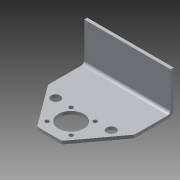
# Autodesk Inventor part: bracket for PG-71
Saved by Autodesk Inventor 2013 (Build 170138000, 138)
## iProperties
Created: 2013-02-02
Part Number: bracket for PG-71
Material: Aluminum 6061
Document SubType Name: Sheet Metal
Designer: aslane
Density: 1 g/cm^3
Sheet Metal Rule: Default
Author: aslane
Autodesk Inventor part; units mm, degrees
ref_plane "YZ Plane" through (0, 0, 0) normal (1, 0, 0) x (0, 1, 0)
ref_plane "XZ Plane" through (0, 0, 0) normal (0, 1, 0) x (-1, 0, 0)
ref_plane "XY Plane" through (0, 0, 0) normal (0, 0, 1) x (1, 0, 0)
sketch "Sketch1" plane through (0, 0, 0) normal (0, 1, 0) x (-1, 0, 0)
  line L0 (30.798, 43.1648) -> (0.6237, 2.4295)
  arc A0 (0.6237, 2.4295) -> (0, 0.5397) centre (3.175, 0.5397) ccw
  line L1 (0, 0.5397) -> (0, 0)
  line L2 (0, 0) -> (88.9, 0)
  line L3 (88.9, 0) -> (88.9, 0.5397)
  arc A1 (88.9, 0.5397) -> (88.2763, 2.4295) centre (85.725, 0.5397) ccw
  line L4 (88.2763, 2.4295) -> (58.102, 43.1648)
  arc A2 (58.102, 43.1648) -> (55.5507, 44.45) centre (55.5507, 41.275) ccw
  line L5 (55.5507, 44.45) -> (33.3493, 44.45)
  arc A3 (33.3493, 44.45) -> (30.798, 43.1648) centre (33.3493, 41.275) ccw
  circle A4 centre (15.875, 9.525) radius 4.7625
  circle A5 centre (44.45, 22.225) radius 13.0556
  circle A6 centre (56.8248, 34.5998) radius 2.1463
  circle A7 centre (56.8248, 9.8502) radius 2.1463
  circle A8 centre (32.0752, 9.8502) radius 2.1463
  circle A9 centre (32.0752, 34.5998) radius 2.1463
  circle A10 centre (73.025, 9.525) radius 4.7625
  line L6 (0, 0) -> (0, -38.8112)
  line L7 (0, -38.8112) -> (88.9, -38.8112)
  line L8 (88.9, -38.8112) -> (88.9, 0)
extrude "Plate1" add sketch "Sketch1" along normal blind 3.175
sketch "Sketch3" plane through (-88.9, 25.4, -41.275) normal (0, 0, 1) x (1, 0, 0)
  line L0 (0, -19.05) -> (88.9, -19.05)
  line L1 (88.9, 0) -> (88.9, -19.05)
  line L2 (88.9, 0) -> (0, 0)
  line L3 (0, 0) -> (0, -19.05)
  line L4 (88.9, -9.525) -> (85.852, -9.525)
  line L5 (88.9, -9.525) -> (82.55, -9.525)
  circle A0 centre (82.55, -9.525) radius 3.302
  line L6 (44.45, -19.05) -> (44.45, 0)
  circle A1 centre (6.35, -9.525) radius 3.302
  line L7 (61.0352, 0) -> (61.0352, 14.605)
  line L8 (61.0352, 14.605) -> (0, 14.605)
  line L9 (0, 14.605) -> (0, 0)
  line L10 (61.0352, 14.605) -> (88.9, 14.605)
  line L11 (88.9, 14.605) -> (88.9, 0)
  line L12 (82.55, -9.525) -> (82.55, 5.08)
  circle A2 centre (82.55, 7.3025) radius 3.302
  circle A3 centre (6.35, 7.3025) radius 3.302
  point P0 (88.9, -25.4)
  dimension "d12" = 3.048
  dimension "d13" = 6.35
  dimension "d14" = 14.605
  dimension "d15" = 14.605
  measures "d12" distance of L4.start L4.end
  measures "d13" distance of L4.start L5.end
  measures "d14" distance of L7.start L7.end
  measures "d15" distance of L12.start L12.end
sketch "Sketch4" plane through (-88.9, 6.35, -41.275) normal (0, 0, 1) x (1, 0, 0)
  line L0 (88.9, 33.655) -> (88.9, 0) projected
  line L1 (0, 33.655) -> (0, 0) projected
  line L2 (0, 26.3525) -> (19.05, 26.3525)
  circle A0 centre (19.05, 26.3525) radius 3.302
  line L3 (88.9, 26.3525) -> (69.85, 26.3525)
  circle A1 centre (69.85, 26.3525) radius 3.302
  point P0 (88.9, -6.35)
  dimension "d21" = 19.05
  dimension "d22" = 6.604
  dimension "d23" = 19.05
  dimension "d24" = 6.604
  constraints: 4 end point, 2 centre point, 2 coincident, 2 point on line, 1 collinear, 1 perpendicular
  measures "d21" distance of L2.start L2.end
  measures "d22" diameter of A0
  measures "d23" distance of L3.start L3.end
  measures "d24" diameter of A1
cut "Cut1" [suppressed]
sketch "Sketch5" plane through (-88.9, 6.35, -41.275) normal (0, 0, 1) x (1, 0, 0)
  circle A0 centre (19.05, 26.3525) radius 3.302 projected
  circle A1 centre (69.85, 26.3525) radius 3.302 projected
  circle A2 centre (82.55, 26.3525) radius 3.302 projected
  circle A3 centre (6.35, 26.3525) radius 3.302 projected
  line L0 (88.9, 33.655) -> (88.9, 0) projected
  line L1 (88.9, 33.655) -> (0, 33.655) projected
  line L2 (0, 33.655) -> (0, 0) projected
  line L3 (88.9, 33.655) -> (88.9, 31.115)
  line L4 (88.9, 31.115) -> (0, 31.115)
  line L5 (6.35, 26.3525) -> (6.35, 23.8125)
  line L6 (82.55, 26.3525) -> (82.55, 23.8125)
  point P0 (88.9, -6.35)
  dimension "d27" = 2.54
  dimension "d28" = 2.54
  constraints: 8 end point, 2 perpendicular, 2 point on line, 1 parallel
  measures "d27" distance of L0.start L3.end
  measures "d28" distance of L5.start L5.end
cut "Cut2" [suppressed]
sketch "Sketch6" plane through (-88.9, 6.35, -41.275) normal (0, 0, 1) x (1, 0, 0)
  circle A0 centre (19.05, 26.3525) radius 3.302
  circle A1 centre (69.85, 26.3525) radius 3.302
  circle A2 centre (82.55, 26.3525) radius 3.302
  circle A3 centre (6.35, 26.3525) radius 3.302
  point P0 (88.9, -6.35)
sketch "Sketch7" plane through (-88.9, 6.35, -41.275) normal (0, 0, 1) x (1, 0, 0)
  line L0 (88.9, 31.115) -> (0, 31.115) projected
  line L1 (0, 31.115) -> (0, 0) projected
  line L2 (88.9, 31.115) -> (88.9, 0) projected
  line L3 (80.0712, 31.115) -> (80.0712, 23.7998)
  line L4 (80.0712, 23.7998) -> (88.9, 23.7998)
  line L5 (88.9, 23.7998) -> (82.55, 23.7998)
  circle A0 centre (82.55, 23.7998) radius 3.302
  line L6 (0, 23.7998) -> (6.35, 23.7998)
  circle A1 centre (6.35, 23.7998) radius 3.302
  point P0 (88.9, -6.35)
  dimension "d36" = 7.3152
  dimension "d39" = 6.35
  dimension "d40" = 6.604
  dimension "d41" = 6.35
  dimension "d42" = 6.604
  constraints: 8 end point, 4 point on line, 2 centre point, 2 coincident, 2 perpendicular, 1 collinear
  measures "d36" distance of L3.start L3.end
  measures "d39" distance of L4.end L5.end
  measures "d40" diameter of A0
  measures "d41" distance of L6.start L6.end
  measures "d42" diameter of A1
cut "Cut3" [suppressed]
sketch "Sketch2" plane through (-88.9, 0, -41.275) normal (0, 0, -1) x (-1, 0, 0)
  line L0 (-88.9, 0) -> (0, 0)
  line L1 (0, 0) -> (0, 25.4)
  line L2 (0, 25.4) -> (-88.9, 25.4)
  line L3 (-88.9, 25.4) -> (-88.9, 0)
  constraints: 6 end point, 1 horizontal, 1 perpendicular, 1 vertical
sketch "Sketch9" plane through (-88.9, 0, -35.6362) normal (0, 0, -1) x (-1, 0, 0)
  line L0 (-88.9, 0) -> (0, 0)
  line L1 (0, 0) -> (0, 37.465)
  line L2 (0, 37.465) -> (-88.9, 37.465)
  line L3 (-88.9, 37.465) -> (-88.9, 0)
  constraints: 6 end point, 1 horizontal, 1 perpendicular, 1 vertical
edge flange "Flange2" height 37.465 angle 90 thickness 3.175 bend radius 3.175 thickness toward (0, 0, -1) relief straight relief width 3.175 relief depth 1.5875 edges at (-44.45, 3.175, -38.8112) wall of the first edge with corners at (0, 0, -35.6362) (-88.9, 0, -35.6362) (-88.9, 37.465, -35.6362) (0, 37.465, -35.6362)
bend "Bend5"
corner "Corner2"
sketch "Sketch8" plane through (-88.9, 6.35, -41.275) normal (0, 0, 1) x (1, 0, 0)
  circle A0 centre (6.35, 23.7998) radius 3.302
  circle A1 centre (82.55, 23.7998) radius 3.302
  point P0 (88.9, -6.35)
sketch "Sketch10" plane through (-88.9, 37.465, -38.8112) normal (0, 1, 0) x (1, 0, 0)
  line L0 (88.9, 0) -> (0, 0) projected
  line L1 (0, -3.175) -> (0, 0) projected
  line L2 (88.9, -3.175) -> (0, -3.175) projected
  line L3 (88.9, -3.175) -> (88.9, 0) projected
  point P0 (88.9, -38.8112)
extrude "Extrusion1" add sketch "Sketch10" along normal blind 5.2324
equation "\"d25\" = Thickness"
equation "\"d29\" = Thickness"
equation "\"d43\" = Thickness"
equation "\"d52\" = BendReliefWidth"
equation "\"d53\" = BendReliefDepth"
equation "\"d54\" = MinimumRemnant"
equation "\"d55\" = BendRadius"
equation "\"d58\" = BendRadius"
equation "\"d59\" = CornerReliefSize"
equation "\"d60\" = GapSize"
equation "\"d61\" = JacobiRadiusSize"
equation "\"BendRadius\" = Thickness"
equation "\"BendReliefWidth\" = Thickness"
equation "\"BendReliefDepth\" = 0.5 * Thickness"
equation "\"CornerReliefSize\" = 4 * Thickness"
equation "\"MinimumRemnant\" = 2 * Thickness"
equation "\"TransitionRadius\" = BendRadius"
equation "\"JacobiRadiusSize\" = BendRadius"
equation "\"GapSize\" = Thickness"
equation "\"d1\" = BendRadius"
equation "\"Thickness\" = 3.175"
body "Solid1"
